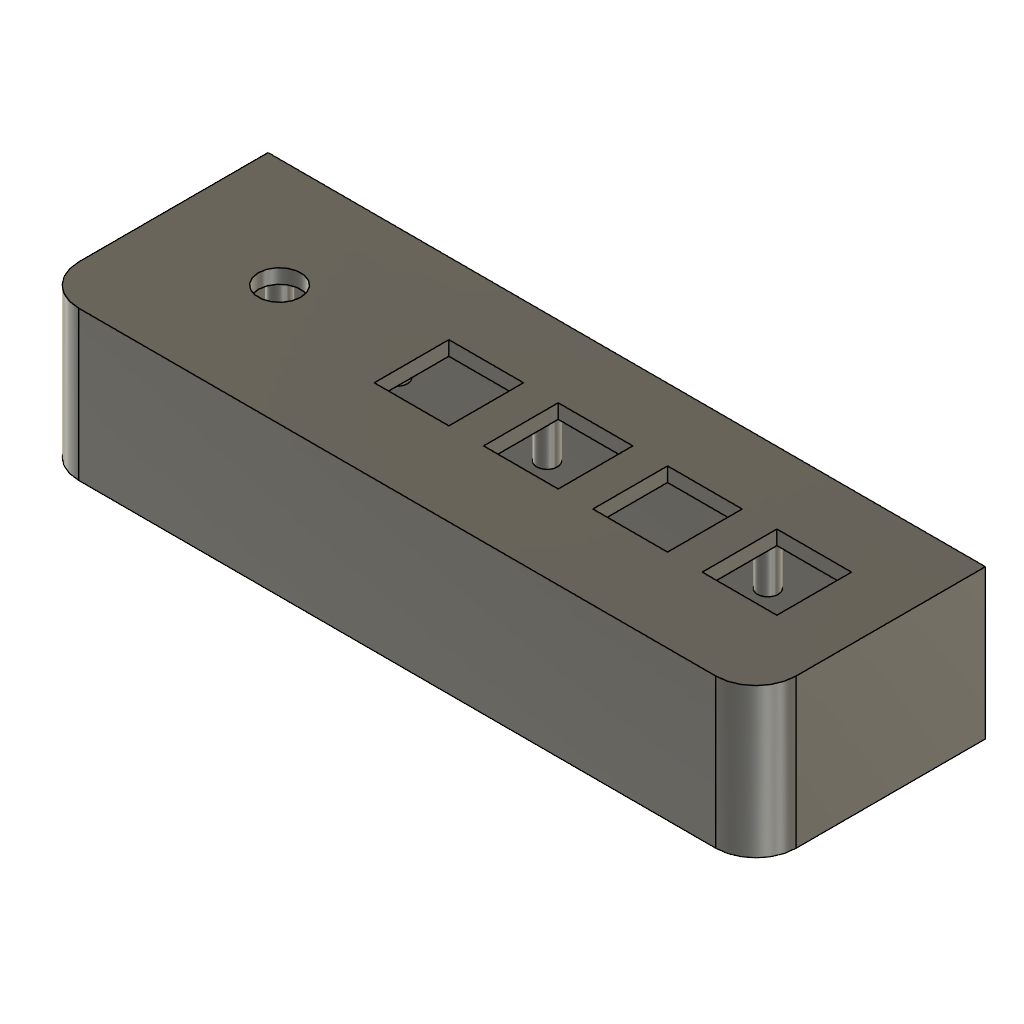
coin-module (Autodesk Fusion 360 design; units mm, degrees)
part number: 2026-10-03-20-53-07-038
Autodesk Fusion 360 part; units mm, degrees
sketch "Esquisse1" plane through (0, 0, 0) normal (0, 0, 1) x (1, 0, 0)
  line L0 (62.5, 20) -> (-62.5, 20)
  line L1 (-62.5, 20) -> (-62.5, -20)
  line L2 (-62.5, -20) -> (62.5, -20)
  line L3 (62.5, -20) -> (62.5, 20)
  line L4 (62.5, 20) -> (-62.5, -20) construction
  line L5 (-62.5, 20) -> (62.5, -20) construction
  dimension "d26" = 125
  dimension "d27" = 40
  constraint horizontal L0
  constraint perpendicular L0 L1
  constraint parallel L0 L2
  constraint parallel L1 L3
  constraint coincident L4 origin
  constraint coincident L5 origin
  measures "d26" distance of L1.end L2.end
  measures "d27" distance of L0.end L1.end
extrude "Extrusion1" add sketch "Esquisse1" along normal blind 26
fillet "Congé1" radius 7 2 edges at (-62.5, -20, 13) (62.5, -20, 13)
shell "Coque1" thickness 2.5 removed faces 1 at (18.5, 6.6667, 0)
sketch "Esquisse2" plane through (0, 0, 26) normal (0, 0, 1) x (-1, 0, 0)
  arc A0 (-55.5, 20) -> (-62.5, 13) centre (-55.5, 13) ccw
  line L0 (-62.5, 13) -> (-62.5, -20)
  line L1 (-62.5, -20) -> (62.5, -20)
  line L2 (62.5, -20) -> (62.5, 13)
  arc A1 (62.5, 13) -> (55.5, 20) centre (55.5, 13) ccw
  line L3 (55.5, 20) -> (-55.5, 20)
  line L4 (5.5, 5.5) -> (18.5, 5.5)
  line L5 (18.5, 5.5) -> (18.5, -7.5)
  line L6 (18.5, -7.5) -> (5.5, -7.5)
  line L7 (5.5, -7.5) -> (5.5, 5.5)
  line L8 (5.5, 5.5) -> (18.5, -7.5) construction
  line L9 (18.5, 5.5) -> (5.5, -7.5) construction
  point P0 (12, -1)
  dimension "d33" = 13
  dimension "d34" = 13
  dimension "d36" = 21
  dimension "d37" = 50.5
  constraint horizontal L4
  constraint perpendicular L4 L5
  constraint parallel L4 L6
  constraint parallel L5 L7
  constraint coincident L8 P0
  constraint coincident L9 P0
  measures "d33" distance of L5.end L6.end
  measures "d34" distance of L4.end L5.end
  measures "d36" distance of L3 P0
  measures "d37" distance of L2 P0
extrude "Extrusion2" cut sketch "Esquisse2" against normal blind 2.5 contours L4 L5 L6 L7
pattern_linear "Réseau R1" count 4 spacing 19.05 along (1, 0, 0) of "Extrusion2"
sketch "Esquisse4" plane through (0, 0, 26) normal (0, 0, 1) x (-1, 0, 0)
  line L0 (-38.65, 5.5) -> (-38.65, -7.5)
  line L1 (-38.65, -7.5) -> (-51.65, -7.5)
  line L2 (-51.65, -7.5) -> (-51.65, 5.5)
  line L3 (-51.65, 5.5) -> (-38.65, 5.5)
  line L4 (-19.6, 5.5) -> (-19.6, -7.5)
  line L5 (-19.6, -7.5) -> (-32.6, -7.5)
  line L6 (-32.6, -7.5) -> (-32.6, 5.5)
  line L7 (-32.6, 5.5) -> (-19.6, 5.5)
  line L8 (-0.55, 5.5) -> (-0.55, -7.5)
  line L9 (-0.55, -7.5) -> (-13.55, -7.5)
  line L10 (-13.55, -7.5) -> (-13.55, 5.5)
  line L11 (-13.55, 5.5) -> (-0.55, 5.5)
  line L12 (18.5, 5.5) -> (18.5, -7.5)
  line L13 (18.5, -7.5) -> (5.5, -7.5)
  line L14 (5.5, -7.5) -> (5.5, 5.5)
  line L15 (5.5, 5.5) -> (18.5, 5.5)
  arc A0 (-55.5, 20) -> (-62.5, 13) centre (-55.5, 13) ccw
  line L16 (-62.5, 13) -> (-62.5, -20)
  line L17 (-62.5, -20) -> (62.5, -20)
  line L18 (62.5, -20) -> (62.5, 13)
  arc A1 (62.5, 13) -> (55.5, 20) centre (55.5, 13) ccw
  line L19 (55.5, 20) -> (-55.5, 20)
  circle A2 centre (41.5, -1) radius 3.7
  dimension "d45" = 7.4
  dimension "d46" = 21
  dimension "d47" = 21
  measures "d45" diameter of A2
  measures "d46" distance of L19 A2.centre
  measures "d47" distance of L18 A2.centre
extrude "Extrusion3" cut sketch "Esquisse4" against normal blind 2.5 contours A2
sketch "Esquisse5" plane through (0, 0, 23.5) normal (0, 0, -1) x (1, 0, 0)
  circle A0 centre (-41.5, -1) radius 3.7
  line L0 (38.65, -7.5) -> (38.65, 5.5)
  line L1 (38.65, 5.5) -> (51.65, 5.5)
  line L2 (51.65, 5.5) -> (51.65, -7.5)
  line L3 (51.65, -7.5) -> (38.65, -7.5)
  line L4 (19.6, -7.5) -> (19.6, 5.5)
  line L5 (19.6, 5.5) -> (32.6, 5.5)
  line L6 (32.6, 5.5) -> (32.6, -7.5)
  line L7 (32.6, -7.5) -> (19.6, -7.5)
  line L8 (0.55, -7.5) -> (0.55, 5.5)
  line L9 (0.55, 5.5) -> (13.55, 5.5)
  line L10 (13.55, 5.5) -> (13.55, -7.5)
  line L11 (13.55, -7.5) -> (0.55, -7.5)
  line L12 (-18.5, -7.5) -> (-18.5, 5.5)
  line L13 (-18.5, 5.5) -> (-5.5, 5.5)
  line L14 (-5.5, 5.5) -> (-5.5, -7.5)
  line L15 (-5.5, -7.5) -> (-18.5, -7.5)
  arc A1 (60, 13) -> (55.5, 17.5) centre (55.5, 13) ccw
  line L16 (55.5, 17.5) -> (-55.5, 17.5)
  arc A2 (-55.5, 17.5) -> (-60, 13) centre (-55.5, 13) ccw
  line L17 (-60, 13) -> (-60, -17.5)
  line L18 (-60, -17.5) -> (60, -17.5)
  line L19 (60, -17.5) -> (60, 13)
  circle A3 centre (-2.675, 6.75) radius 1.8
  line L20 (62.5, 13) -> (62.5, -20)
  line L21 (-62.5, -20) -> (-62.5, 13)
  line L22 (62.5, -20) -> (-62.5, -20)
  circle A4 centre (35.825, -8.75) radius 1.8
  circle A5 centre (35.825, 6.75) radius 1.8
  line L23 (-55.5, 20) -> (55.5, 20)
  circle A6 centre (-2.6369, -8.75) radius 1.8
  dimension "d50" = 3.6
  dimension "d52" = 59.825
  dimension "d54" = 3.6
  dimension "d56" = 98.325
  dimension "d57" = 3.6
  dimension "d59" = 28.75
  dimension "d60" = 13.25
  dimension "d61" = 13.25
  dimension "d62" = 3.6
  dimension "d63" = 28.75
  dimension "d64" = 98.325
  measures "d50" diameter of A3
  measures "d52" distance of A3.centre L21
  measures "d54" diameter of A4
  measures "d56" distance of L21 A4.centre
  measures "d57" diameter of A5
  measures "d59" distance of A4.centre L23
  measures "d60" distance of A5.centre L23
  measures "d61" distance of A3.centre L23
  measures "d62" diameter of A6
  measures "d63" distance of L23 A6.centre
  measures "d64" distance of L21 A5.centre
extrude "Extrusion4" add sketch "Esquisse5" along normal blind 8.5 contours A3 | A4 | A5 | A6
sketch "Esquisse6" plane through (0, 0, 23.5) normal (0, 0, -1) x (1, 0, 0)
  circle A0 centre (35.825, -8.75) radius 1.8
  circle A1 centre (-2.675, 6.75) radius 1.8
  circle A2 centre (-2.6369, -8.75) radius 1.8
  circle A3 centre (-41.5, -1) radius 3.7
  line L0 (38.65, -7.5) -> (38.65, 5.5)
  line L1 (38.65, 5.5) -> (51.65, 5.5)
  line L2 (51.65, 5.5) -> (51.65, -7.5)
  line L3 (51.65, -7.5) -> (38.65, -7.5)
  line L4 (19.6, -7.5) -> (19.6, 5.5)
  line L5 (19.6, 5.5) -> (32.6, 5.5)
  line L6 (32.6, 5.5) -> (32.6, -7.5)
  line L7 (32.6, -7.5) -> (19.6, -7.5)
  line L8 (0.55, -7.5) -> (0.55, 5.5)
  line L9 (0.55, 5.5) -> (13.55, 5.5)
  line L10 (13.55, 5.5) -> (13.55, -7.5)
  line L11 (13.55, -7.5) -> (0.55, -7.5)
  line L12 (-18.5, -7.5) -> (-18.5, 5.5)
  line L13 (-18.5, 5.5) -> (-5.5, 5.5)
  line L14 (-5.5, 5.5) -> (-5.5, -7.5)
  line L15 (-5.5, -7.5) -> (-18.5, -7.5)
  arc A4 (60, 13) -> (55.5, 17.5) centre (55.5, 13) ccw
  line L16 (55.5, 17.5) -> (-55.5, 17.5)
  arc A5 (-55.5, 17.5) -> (-60, 13) centre (-55.5, 13) ccw
  line L17 (-60, 13) -> (-60, -17.5)
  line L18 (-60, -17.5) -> (60, -17.5)
  line L19 (60, -17.5) -> (60, 13)
  circle A6 centre (35.825, 6.75) radius 1.8
  circle A7 centre (-31.25, -11.25) radius 1.8
  line L20 (-62.5, -20) -> (-62.5, 13)
  line L21 (-55.5, 20) -> (55.5, 20)
  dimension "d67" = 3.6
  dimension "d68" = 31.25
  dimension "d69" = 31.25
  measures "d67" diameter of A7
  measures "d68" distance of A7.centre L20
  measures "d69" distance of A7.centre L21
sketch "Esquisse7" plane through (0, 0, 23.5) normal (0, 0, -1) x (1, 0, 0)
  circle A0 centre (-31.25, 9.25) radius 1.8
  line L0 (-55.5, 20) -> (55.5, 20)
  line L1 (-62.5, -20) -> (-62.5, 13)
  dimension "d70" = 3.6
  dimension "d71" = 10.75
  dimension "d72" = 31.25
  measures "d70" diameter of A0
  measures "d71" distance of A0.centre L0
  measures "d72" distance of A0.centre L1
sketch "Esquisse10" plane through (0, 0, 23.5) normal (0, 0, -1) x (1, 0, 0)
  circle A0 centre (-51.75, -11.25) radius 1.8
  line L0 (-55.5, 20) -> (55.5, 20)
  line L1 (-62.5, -20) -> (-62.5, 13)
  dimension "d77" = 3.6
  dimension "d78" = 31.25
  dimension "d79" = 10.75
  measures "d77" diameter of A0
  measures "d78" distance of A0.centre L0
  measures "d79" distance of A0.centre L1
sketch "Esquisse11" plane through (0, 0, 23.5) normal (0, 0, -1) x (1, 0, 0)
  circle A0 centre (-51.75, 9.25) radius 1.8
  line L0 (-62.5, -20) -> (-62.5, 13)
  line L1 (-55.5, 20) -> (55.5, 20)
  dimension "d80" = 3.6
  dimension "d81" = 10.75
  dimension "d82" = 10.75
  measures "d80" diameter of A0
  measures "d81" distance of A0.centre L0
  measures "d82" distance of A0.centre L1
extrude "Extrusion5" add sketch "Esquisse6" sketch "Esquisse10" sketch "Esquisse11" sketch "Esquisse7" along normal blind 11.5 contours A7 of sketch 2 of sketch 3 of sketch 4
sketch "Esquisse12" plane through (0, 0, 15) normal (0, 0, -1) x (1, 0, 0)
  circle A0 centre (35.825, -8.75) radius 1.8
  circle A1 centre (35.825, -8.75) radius 0.8
  dimension "d85" = 1.6
  constraint concentric A0 A1
  measures "d85" diameter of A1
sketch "Esquisse13" plane through (0, 0, 15) normal (0, 0, -1) x (1, 0, 0)
  circle A0 centre (35.825, 6.75) radius 1.8
  circle A1 centre (35.825, 6.75) radius 0.8
  dimension "d86" = 1.6
  constraint concentric A0 A1
  measures "d86" diameter of A1
sketch "Esquisse14" plane through (0, 0, 15) normal (0, 0, -1) x (1, 0, 0)
  circle A0 centre (-2.6369, -8.75) radius 1.8
  circle A1 centre (-2.6369, -8.75) radius 0.8
  dimension "d87" = 1.6
  constraint concentric A0 A1
  measures "d87" diameter of A1
sketch "Esquisse15" plane through (0, 0, 15) normal (0, 0, -1) x (1, 0, 0)
  circle A0 centre (-2.675, 6.75) radius 1.8
  circle A1 centre (-2.675, 6.75) radius 0.8
  dimension "d88" = 1.6
  constraint concentric A0 A1
  measures "d88" diameter of A1
sketch "Esquisse16" plane through (0, 0, 12) normal (0, 0, -1) x (1, 0, 0)
  circle A0 centre (-31.25, -11.25) radius 1.8
  circle A1 centre (-31.25, -11.25) radius 0.8
  dimension "d89" = 1.6
  constraint concentric A0 A1
  measures "d89" diameter of A1
sketch "Esquisse17" plane through (0, 0, 12) normal (0, 0, -1) x (1, 0, 0)
  circle A0 centre (-31.25, 9.25) radius 1.8
  circle A1 centre (-31.25, 9.25) radius 0.8
  dimension "d90" = 1.6
  constraint concentric A0 A1
  measures "d90" diameter of A1
sketch "Esquisse18" plane through (0, 0, 12) normal (0, 0, -1) x (1, 0, 0)
  circle A0 centre (-51.75, -11.25) radius 1.8
  circle A1 centre (-51.75, -11.25) radius 0.8
  dimension "d91" = 1.6
  constraint concentric A0 A1
  measures "d91" diameter of A1
sketch "Esquisse19" plane through (0, 0, 12) normal (0, 0, -1) x (1, 0, 0)
  circle A0 centre (-51.75, 9.25) radius 1.8
  circle A1 centre (-51.75, 9.25) radius 0.8
  dimension "d92" = 1.6
  constraint concentric A0 A1
  measures "d92" diameter of A1
extrude "Extrusion6" cut sketch "Esquisse12" sketch "Esquisse13" sketch "Esquisse14" sketch "Esquisse15" against normal blind 6 contours A1 of sketch 2 contours A1 of sketch 3 contours A1 of sketch 4 contours A1
extrude "Extrusion7" cut sketch "Esquisse18" sketch "Esquisse19" sketch "Esquisse17" sketch "Esquisse16" against normal blind 6 contours A1 of sketch 2 contours A1 of sketch 3 contours A1 of sketch 4 contours A1
equation "l_module = 125 mm"
equation "h_test = 40 mm"
equation "ep_module = 26 mm"
equation "r_module = 7 mm"
equation "ep_paroi = 2.5 mm"
equation "y_commandes = 21 mm"
equation "x_molette = 21 mm"
equation "x_touche1 = 50.5 mm"
equation "pas_touche = 19.05 mm"
equation "fen_switch = 13 mm"
equation "l_neokey = 76.5 mm"
equation "w_neokey = 21.5 mm"
equation "marge_switch = 9.675 mm"
equation "x_neokey = 40.825 mm"
equation "y_neokey = 10.25 mm"
equation "trou_nk_x = 19 mm"
equation "trou_nk_y = 3 mm"
equation "prof_neokey = 11 mm"
equation "c_encodeur = 25.5 mm"
equation "trou_enc = 2.5 mm"
equation "prof_encodeur = 14 mm"
equation "d_bague = 7 mm"
equation "jeu_bague = 0.2 mm"
equation "d_plot = 3.6 mm"
equation "d_pilote = 1.6 mm"
equation "d26 = l_module"
equation "d27 = h_test"
equation "d28 = ep_module"
equation "d31 = r_module"
equation "d32 = ep_paroi"
equation "d33 = fen_switch"
equation "d34 = fen_switch"
equation "d36 = y_commandes"
equation "d37 = x_touche1"
equation "d38 = -ep_paroi"
equation "d42 = pas_touche"
equation "d45 = d_bague + 2 * jeu_bague"
equation "d46 = y_commandes"
equation "d47 = x_molette"
equation "d48 = -ep_paroi"
equation "d50 = d_plot"
equation "d52 = x_neokey + trou_nk_x"
equation "d54 = d_plot"
equation "d56 = x_neokey + l_neokey - trou_nk_x"
equation "d57 = d_plot"
equation "d59 = y_neokey + w_neokey - trou_nk_y"
equation "d60 = y_neokey + trou_nk_y"
equation "d61 = y_neokey + trou_nk_y"
equation "d62 = d_plot"
equation "d63 = y_neokey + w_neokey - trou_nk_y"
equation "d64 = x_neokey + l_neokey - trou_nk_x"
equation "d65 = prof_neokey - ep_paroi"
equation "d67 = d_plot"
equation "d68 = x_molette + ( c_encodeur / 2 - trou_enc )"
equation "d69 = y_commandes + ( c_encodeur / 2 - trou_enc )"
equation "d70 = d_plot"
equation "d71 = y_commandes - ( c_encodeur / 2 - trou_enc )"
equation "d72 = x_molette + ( c_encodeur / 2 - trou_enc )"
equation "d77 = d_plot"
equation "d78 = y_commandes + ( c_encodeur / 2 - trou_enc )"
equation "d79 = x_molette - ( c_encodeur / 2 - trou_enc )"
equation "d80 = d_plot"
equation "d81 = x_molette - ( c_encodeur / 2 - trou_enc )"
equation "d82 = y_commandes - ( c_encodeur / 2 - trou_enc )"
equation "d83 = prof_encodeur - ep_paroi"
equation "d85 = d_pilote"
equation "d86 = d_pilote"
equation "d87 = d_pilote"
equation "d88 = d_pilote"
equation "d89 = d_pilote"
equation "d90 = d_pilote"
equation "d91 = d_pilote"
equation "d92 = d_pilote"
